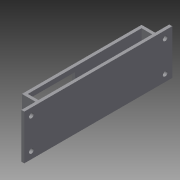
# Autodesk Inventor part: Autonomous - Phone Case V2
Saved by Autodesk Inventor 2015 (Build 190159000, 159)
## iProperties
Created: 2015-05-13
Part Number: Autonomous - Phone Case V2
Material: Generic
Document SubType Name: Modeling
Designer: 166189
Density: 1 g/cm^3
Appearance: Default
Author: 166189
Autodesk Inventor part; units mm, degrees
ref_plane "YZ Plane" through (0, 0, 0) normal (1, 0, 0) x (0, 1, 0)
ref_plane "XZ Plane" through (0, 0, 0) normal (0, 1, 0) x (-1, 0, 0)
ref_plane "XY Plane" through (0, 0, 0) normal (0, 0, 1) x (1, 0, 0)
sketch "Sketch1" plane through (0, 0, 0) normal (0, 1, 0) x (-1, 0, 0)
  line L0 (0, 0) -> (0, -128.905)
  line L1 (0, -128.905) -> (17.78, -128.905)
  line L2 (17.78, -128.905) -> (17.78, 0)
  line L3 (17.78, 0) -> (0, 0)
  dimension "d0" = 128.905
  dimension "d1" = 17.78
  constraints: 8 end point, 3 perpendicular, 1 vertical
  measures "d0" distance of L0.start L0.end
  measures "d1" distance of L0.end L1.end
extrude "Extrusion1" add sketch "Sketch1" along normal blind 48.26
sketch "Sketch2" plane through (0, 48.26, 0) normal (0, 1, 0) x (1, 0, 0)
  line L0 (0, 0) -> (0, 3.175)
  line L1 (0, 0) -> (0, 128.905) projected
  line L2 (0, 3.175) -> (-3.175, 3.175)
  line L3 (-3.175, 3.175) -> (-3.175, 125.73)
  line L4 (-3.175, 125.73) -> (-14.605, 125.73)
  line L5 (-14.605, 125.73) -> (-14.605, 3.175)
  line L6 (-14.605, 3.175) -> (-3.175, 3.175)
  dimension "d4" = 3.175
  dimension "d5" = 3.175
  dimension "d6" = 122.555
  dimension "d7" = 11.43
  constraints: 12 end point, 5 perpendicular, 2 point on line
  measures "d4" distance of L0.start L0.end
  measures "d5" distance of L0.end L2.end
  measures "d6" distance of L2.end L3.end
  measures "d7" distance of L3.end L4.end
extrude "Extrusion2" cut sketch "Sketch2" against normal blind 43.18
sketch "Sketch3" plane through (-17.78, 0, -128.905) normal (-1, 0, 0) x (0, 0, 1)
  line L0 (128.905, 0) -> (125.73, 0)
  line L1 (128.905, 0) -> (0, 0) projected
  line L2 (125.73, 0) -> (125.73, 5.08)
  line L3 (125.73, 5.08) -> (74.93, 5.08)
  line L4 (3.175, 5.08) -> (125.73, 5.08) projected
  line L5 (74.93, 5.08) -> (74.93, 43.18)
  line L6 (0, 48.26) -> (128.905, 48.26) projected
  line L7 (74.93, 43.18) -> (125.73, 43.18)
  line L8 (125.73, 48.26) -> (125.73, 5.08) projected
  dimension "d10" = 3.175
  dimension "d11" = 5.08
  dimension "d12" = 50.8
  dimension "d13" = 38.1
  constraints: 10 end point, 3 perpendicular, 3 point on line
  measures "d10" distance of L0.start L0.end
  measures "d11" distance of L0.end L2.end
  measures "d12" distance of L2.end L3.end
  measures "d13" distance of L3.end L5.end
extrude "Extrusion3" cut sketch "Sketch3" against normal blind 5.08
sketch "Sketch4" plane through (-17.78, 0, 0) normal (0, 0, 1) x (1, 0, 0)
  line L0 (17.78, 0) -> (14.605, 0)
  line L1 (0, 0) -> (17.78, 0) projected
  line L2 (14.605, 0) -> (14.605, 48.26)
  line L3 (17.78, 48.26) -> (0, 48.26) projected
  line L4 (17.78, 48.26) -> (17.78, 0)
  line L5 (17.78, 0) -> (17.78, 48.26) projected
  dimension "d16" = 3.175
  constraints: 6 end point, 2 point on line, 1 collinear, 1 perpendicular
  measures "d16" distance of L0.start L0.end
extrude "Extrusion4" add sketch "Sketch4" along normal blind 15.24
sketch "Sketch5" plane through (-3.175, 0, 0) normal (-1, 0, 0) x (0, 0, 1)
  line L0 (15.24, 48.26) -> (7.62, 48.26)
  line L1 (0, 48.26) -> (15.24, 48.26) projected
  line L2 (7.62, 48.26) -> (7.62, 40.64)
  circle A0 centre (7.62, 40.64) radius 2.54
  line L3 (15.24, 0) -> (7.62, 0)
  line L4 (0, 0) -> (15.24, 0) projected
  line L5 (7.62, 0) -> (7.62, 7.62)
  circle A1 centre (7.62, 7.62) radius 2.54
  dimension "d19" = 7.62
  dimension "d20" = 7.62
  dimension "d21" = 5.08
  dimension "d22" = 7.62
  dimension "d23" = 7.62
  dimension "d24" = 5.08
  constraints: 8 end point, 2 centre point, 2 coincident, 2 midpoint, 2 perpendicular
  measures "d19" distance of L0.start L0.end
  measures "d20" distance of L0.end L2.end
  measures "d21" diameter of A0
  measures "d22" distance of L3.start L3.end
  measures "d23" distance of L3.end L5.end
  measures "d24" diameter of A1
extrude "Extrusion5" cut sketch "Sketch5" against normal blind 15.24
sketch "Sketch6" plane through (0, 0, -128.905) normal (0, 0, -1) x (-1, 0, 0)
  line L0 (0, 48.26) -> (3.175, 48.26)
  line L1 (3.175, 48.26) -> (3.175, 0)
  line L2 (3.175, 48.26) -> (3.175, 0) projected
  line L3 (3.175, 0) -> (0, 0)
  line L4 (0, 0) -> (0, 48.26)
  line L5 (0, 0) -> (0, 48.26) projected
  dimension "d27" = 3.175
  constraints: 8 end point, 2 collinear, 1 horizontal, 1 perpendicular
  measures "d27" distance of L0.start L0.end
extrude "Extrusion6" add sketch "Sketch6" along normal blind 15.24
sketch "Sketch7" plane through (-3.175, 0, -128.905) normal (-1, 0, 0) x (0, 0, 1)
  line L0 (-15.24, 48.26) -> (-15.24, 40.64)
  line L1 (-15.24, 48.26) -> (-15.24, 0) projected
  line L2 (-15.24, 40.64) -> (-7.62, 40.64)
  line L3 (-15.24, 0) -> (-7.62, 0)
  line L4 (0, 0) -> (-15.24, 0) projected
  line L5 (-7.62, 0) -> (-7.62, 7.62)
  circle A0 centre (-7.62, 7.62) radius 2.54
  circle A1 centre (-7.62, 40.64) radius 2.54
  point P0 (128.905, 0)
  dimension "d30" = 7.62
  dimension "d31" = 7.62
  dimension "d32" = 7.62
  dimension "d33" = 7.62
  dimension "d34" = 5.08
  dimension "d35" = 5.08
  constraints: 8 end point, 2 centre point, 2 coincident, 2 perpendicular, 1 midpoint, 1 point on line
  measures "d30" distance of L0.start L0.end
  measures "d31" distance of L0.end L2.end
  measures "d32" distance of L1.end L3.end
  measures "d33" distance of L3.end L5.end
  measures "d34" diameter of A0
  measures "d35" diameter of A1
extrude "Extrusion7" cut sketch "Sketch7" against normal blind 15.24
body "Solid1"
